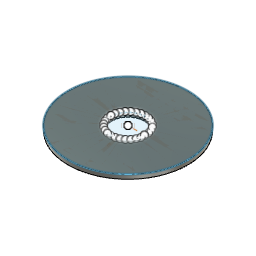
Untitled v1 (Autodesk Fusion 360 design; units mm, degrees)
Autodesk Fusion 360 part; units mm, degrees
sketch "Sketch2" plane through (0, 0, 0) normal (0, 0, 1) x (1, 0, 0)
  circle A0 centre (0, 0) radius 139.7
  dimension "d37" = 279.4
  constraint coincident A0.centre origin
  measures "d37" diameter of A0
sketch "Sketch1" plane through (0, 0, 0) normal (0, 0, 1) x (1, 0, 0)
  circle A0 centre (0, 0) radius 139.7
  line L0 (7.734, 37.3068) -> (8.2303, 39.481)
  line L1 (9.2198, 36.9676) -> (9.7161, 39.1418)
  line L2 (15.8416, 34.6505) -> (16.8092, 36.6597)
  line L3 (17.2146, 33.9892) -> (18.1823, 35.9985)
  line L4 (23.1548, 30.2567) -> (24.5452, 32.0003)
  line L5 (24.3463, 29.3065) -> (25.7367, 31.05)
  line L6 (29.3069, 24.3457) -> (31.0505, 25.7362)
  line L7 (30.2571, 23.1542) -> (32.0007, 24.5447)
  line L8 (33.9895, 17.214) -> (35.9988, 18.1816)
  line L9 (34.6507, 15.841) -> (36.66, 16.8086)
  line L10 (36.9678, 9.2192) -> (39.142, 9.7154)
  line L11 (37.3069, 7.7334) -> (39.4811, 8.2296)
  line L12 (-0.7493, 40.3155) -> (-0.7493, 38.0926)
  line L13 (0.7493, 40.3155) -> (0.7493, 38.0926)
  arc A1 (15.8416, 34.6505) -> (9.2198, 36.9676) centre (0, 0) ccw
  arc A2 (23.1548, 30.2567) -> (17.2146, 33.9892) centre (0, 0) ccw
  arc A3 (18.1791, 35.992) -> (16.8061, 36.6532) centre (0, 0) ccw
  arc A4 (25.7322, 31.0444) -> (24.5407, 31.9946) centre (0, 0) ccw
  arc A5 (31.9951, 24.5402) -> (31.0449, 25.7317) centre (0, 0) ccw
  arc A6 (29.3069, 24.3457) -> (24.3463, 29.3065) centre (0, 0) ccw
  arc A7 (36.6535, 16.8054) -> (35.9923, 18.1785) centre (0, 0) ccw
  arc A8 (33.9895, 17.214) -> (30.2571, 23.1542) centre (0, 0) ccw
  arc A9 (36.9678, 9.2192) -> (34.6507, 15.841) centre (0, 0) ccw
  arc A10 (39.4741, 8.228) -> (39.135, 9.7138) centre (0, 0) ccw
  arc A11 (38.0926, 0.7493) -> (37.3069, 7.7334) centre (0, 0) ccw
  line L14 (38.0926, 0.7493) -> (40.3155, 0.7493)
  line L15 (38.0926, -0.7493) -> (40.3155, -0.7493)
  arc A12 (9.7145, 39.1348) -> (8.2287, 39.4739) centre (0, 0) ccw
  line L16 (7.734, -37.3068) -> (8.2303, -39.481)
  arc A13 (8.2287, -39.4739) -> (9.7145, -39.1348) centre (0, 0) ccw
  line L17 (9.2198, -36.9676) -> (9.7161, -39.1418)
  arc A14 (9.2198, -36.9676) -> (15.8416, -34.6505) centre (0, 0) ccw
  line L18 (15.8416, -34.6505) -> (16.8092, -36.6597)
  arc A15 (16.8061, -36.6532) -> (18.1791, -35.992) centre (0, 0) ccw
  line L19 (17.2146, -33.9892) -> (18.1823, -35.9985)
  arc A16 (17.2146, -33.9892) -> (23.1548, -30.2567) centre (0, 0) ccw
  line L20 (23.1548, -30.2567) -> (24.5452, -32.0003)
  arc A17 (24.5407, -31.9946) -> (25.7322, -31.0444) centre (0, 0) ccw
  line L21 (24.3463, -29.3065) -> (25.7367, -31.05)
  arc A18 (24.3463, -29.3065) -> (29.3069, -24.3457) centre (0, 0) ccw
  line L22 (29.3069, -24.3457) -> (31.0505, -25.7362)
  arc A19 (31.0449, -25.7317) -> (31.9951, -24.5402) centre (0, 0) ccw
  line L23 (30.2571, -23.1542) -> (32.0007, -24.5447)
  arc A20 (30.2571, -23.1542) -> (33.9895, -17.214) centre (0, 0) ccw
  line L24 (33.9895, -17.214) -> (35.9988, -18.1816)
  arc A21 (35.9923, -18.1785) -> (36.6535, -16.8054) centre (0, 0) ccw
  line L25 (34.6507, -15.841) -> (36.66, -16.8086)
  arc A22 (34.6507, -15.841) -> (36.9678, -9.2192) centre (0, 0) ccw
  line L26 (36.9678, -9.2192) -> (39.142, -9.7154)
  arc A23 (39.135, -9.7138) -> (39.4741, -8.228) centre (0, 0) ccw
  line L27 (37.3069, -7.7334) -> (39.4811, -8.2296)
  arc A24 (37.3069, -7.7334) -> (38.0926, -0.7493) centre (0, 0) ccw
  line L28 (0, 0) -> (38.1, 0) construction
  arc A25 (40.3155, -0.7493) -> (40.3155, 0.7493) centre (0, 0) ccw
  arc A26 (18.1791, 35.992) -> (16.8061, 36.6532) centre (0, 0) ccw
  arc A27 (25.7322, 31.0444) -> (24.5407, 31.9946) centre (0, 0) ccw
  arc A28 (31.9951, 24.5402) -> (31.0449, 25.7317) centre (0, 0) ccw
  arc A29 (39.4741, 8.228) -> (39.135, 9.7138) centre (0, 0) ccw
  arc A30 (36.6535, 16.8054) -> (35.9923, 18.1785) centre (0, 0) ccw
  arc A31 (9.7145, 39.1348) -> (8.2287, 39.4739) centre (0, 0) ccw
  arc A32 (39.135, -9.7138) -> (39.4741, -8.228) centre (0, 0) ccw
  arc A33 (35.9923, -18.1785) -> (36.6535, -16.8054) centre (0, 0) ccw
  arc A34 (31.0449, -25.7317) -> (31.9951, -24.5402) centre (0, 0) ccw
  arc A35 (24.5407, -31.9946) -> (25.7322, -31.0444) centre (0, 0) ccw
  arc A36 (16.8061, -36.6532) -> (18.1791, -35.992) centre (0, 0) ccw
  arc A37 (8.2287, -39.4739) -> (9.7145, -39.1348) centre (0, 0) ccw
  arc A38 (34.6507, -15.841) -> (36.9678, -9.2192) centre (0, 0) ccw
  arc A39 (30.2571, -23.1542) -> (33.9895, -17.214) centre (0, 0) ccw
  arc A40 (24.3463, -29.3065) -> (29.3069, -24.3457) centre (0, 0) ccw
  arc A41 (17.2146, -33.9892) -> (23.1548, -30.2567) centre (0, 0) ccw
  arc A42 (9.2198, -36.9676) -> (15.8416, -34.6505) centre (0, 0) ccw
  arc A43 (-40.3155, 0.7493) -> (-40.3155, -0.7493) centre (0, 0) ccw
  line L29 (-38.0926, -0.7493) -> (-40.3155, -0.7493)
  arc A44 (-38.0926, -0.7493) -> (-37.3069, -7.7334) centre (0, 0) ccw
  line L30 (-37.3069, -7.7334) -> (-39.4811, -8.2296)
  line L31 (-34.6507, -15.841) -> (-36.66, -16.8086)
  arc A45 (-39.4741, -8.228) -> (-39.135, -9.7138) centre (0, 0) ccw
  line L32 (-36.9678, -9.2192) -> (-39.142, -9.7154)
  arc A46 (-36.9678, -9.2192) -> (-34.6507, -15.841) centre (0, 0) ccw
  arc A47 (-36.6535, -16.8054) -> (-35.9923, -18.1785) centre (0, 0) ccw
  line L33 (-33.9895, -17.214) -> (-35.9988, -18.1816)
  arc A48 (-33.9895, -17.214) -> (-30.2571, -23.1542) centre (0, 0) ccw
  line L34 (-30.2571, -23.1542) -> (-32.0007, -24.5447)
  arc A49 (-31.9951, -24.5402) -> (-31.0449, -25.7317) centre (0, 0) ccw
  line L35 (-29.3069, -24.3457) -> (-31.0505, -25.7362)
  arc A50 (-29.3069, -24.3457) -> (-24.3463, -29.3065) centre (0, 0) ccw
  line L36 (-24.3463, -29.3065) -> (-25.7367, -31.05)
  arc A51 (-25.7322, -31.0444) -> (-24.5407, -31.9946) centre (0, 0) ccw
  line L37 (-23.1548, -30.2567) -> (-24.5452, -32.0003)
  arc A52 (-23.1548, -30.2567) -> (-17.2146, -33.9892) centre (0, 0) ccw
  arc A53 (-18.1791, -35.992) -> (-16.8061, -36.6532) centre (0, 0) ccw
  line L38 (-17.2146, -33.9892) -> (-18.1823, -35.9985)
  line L39 (-15.8416, -34.6505) -> (-16.8092, -36.6597)
  arc A54 (-15.8416, -34.6505) -> (-9.2198, -36.9676) centre (0, 0) ccw
  line L40 (-9.2198, -36.9676) -> (-9.7161, -39.1418)
  arc A55 (-9.7145, -39.1348) -> (-8.2287, -39.4739) centre (0, 0) ccw
  line L41 (-7.734, -37.3068) -> (-8.2303, -39.481)
  arc A56 (-15.8416, -34.6505) -> (-9.2198, -36.9676) centre (0, 0) ccw
  arc A57 (-15.8416, -34.6505) -> (-9.2198, -36.9676) centre (0, 0) ccw
  arc A58 (-0.7493, -40.3155) -> (0.7493, -40.3155) centre (0, 0) ccw
  arc A59 (-9.7145, -39.1348) -> (-8.2287, -39.4739) centre (0, 0) ccw
  arc A60 (-0.7493, -40.3155) -> (0, -40.3225) centre (0, 0) ccw
  arc A61 (-9.7145, -39.1348) -> (-8.2287, -39.4739) centre (0, 0) ccw
  arc A62 (-18.1791, -35.992) -> (-16.8061, -36.6532) centre (0, 0) ccw
  arc A63 (-18.1791, -35.992) -> (-16.8061, -36.6532) centre (0, 0) ccw
  arc A64 (-25.7322, -31.0444) -> (-24.5407, -31.9946) centre (0, 0) ccw
  arc A65 (-36.6535, -16.8054) -> (-35.9923, -18.1785) centre (0, 0) ccw
  arc A66 (-39.4741, -8.228) -> (-39.135, -9.7138) centre (0, 0) ccw
  arc A67 (-39.4741, -8.228) -> (-39.135, -9.7138) centre (0, 0) ccw
  arc A68 (-31.9951, -24.5402) -> (-31.0449, -25.7317) centre (0, 0) ccw
  arc A69 (-25.7322, -31.0444) -> (-24.5407, -31.9946) centre (0, 0) ccw
  arc A70 (-23.1548, -30.2567) -> (-17.2146, -33.9892) centre (0, 0) ccw
  arc A71 (-29.3069, -24.3457) -> (-24.3463, -29.3065) centre (0, 0) ccw
  arc A72 (-24.3463, -29.3065) -> (-17.2146, -33.9892) centre (0, 0) ccw
  arc A73 (-33.9895, -17.214) -> (-30.2571, -23.1542) centre (0, 0) ccw
  arc A74 (-36.6535, -16.8054) -> (-35.9923, -18.1785) centre (0, 0) ccw
  arc A75 (-31.9951, -24.5402) -> (-31.0449, -25.7317) centre (0, 0) ccw
  arc A76 (-36.9678, -9.2192) -> (-34.6507, -15.841) centre (0, 0) ccw
  arc A77 (-36.9678, -9.2192) -> (-34.6507, -15.841) centre (0, 0) ccw
  arc A78 (-33.9895, -17.214) -> (-30.2571, -23.1542) centre (0, 0) ccw
  arc A79 (-38.0926, -0.7493) -> (-37.3069, -7.7334) centre (0, 0) ccw
  arc A80 (-38.0926, -0.7493) -> (-37.3069, -7.7334) centre (0, 0) ccw
  arc A81 (-7.734, -37.3068) -> (-0.7493, -38.0926) centre (0, 0) ccw
  arc A82 (-7.734, -37.3068) -> (-0.7493, -38.0926) centre (0, 0) ccw
  arc A83 (0.762, -38.0924) -> (7.734, -37.3068) centre (0, 0) ccw
  arc A84 (-7.734, -37.3068) -> (-0.7493, -38.0926) centre (0, 0) ccw
  arc A85 (0.762, -38.0924) -> (7.734, -37.3068) centre (0, 0) ccw
  line L42 (0.762, -38.0924) -> (0.7493, -40.3155)
  line L43 (-0.7493, -38.0926) -> (-0.7493, -40.3155)
  arc A86 (15.8416, 34.6505) -> (9.2198, 36.9676) centre (0, 0) ccw
  arc A87 (15.8416, 34.6505) -> (9.2198, 36.9676) centre (0, 0) ccw
  arc A88 (23.1548, 30.2567) -> (17.2146, 33.9892) centre (0, 0) ccw
  arc A89 (23.1548, 30.2567) -> (17.2146, 33.9892) centre (0, 0) ccw
  arc A90 (29.3069, 24.3457) -> (24.3463, 29.3065) centre (0, 0) ccw
  arc A91 (29.3069, 24.3457) -> (24.3463, 29.3065) centre (0, 0) ccw
  arc A92 (33.9895, 17.214) -> (30.2571, 23.1542) centre (0, 0) ccw
  arc A93 (33.9895, 17.214) -> (30.2571, 23.1542) centre (0, 0) ccw
  arc A94 (36.9678, 9.2192) -> (34.6507, 15.841) centre (0, 0) ccw
  arc A95 (38.0926, 0.7493) -> (37.3069, 7.7334) centre (0, 0) ccw
  arc A96 (36.9678, 9.2192) -> (34.6507, 15.841) centre (0, 0) ccw
  arc A97 (38.0926, 0.7493) -> (37.3069, 7.7334) centre (0, 0) ccw
  line L44 (-40.3155, 0.7493) -> (-38.0926, 0.7493)
  arc A98 (0, 40.3225) -> (-0.7493, 40.3155) centre (0, 0) ccw
  line L45 (-0.7493, 38.0926) -> (-0.7493, 40.3155)
  arc A99 (-0.7493, 38.0926) -> (-7.734, 37.3068) centre (0, 0) ccw
  line L46 (-7.734, 37.3068) -> (-8.2303, 39.481)
  arc A100 (-8.2287, 39.4739) -> (-9.7145, 39.1348) centre (0, 0) ccw
  line L47 (-9.2198, 36.9676) -> (-9.7161, 39.1418)
  arc A101 (-9.2198, 36.9676) -> (-15.8416, 34.6505) centre (0, 0) ccw
  line L48 (-15.8416, 34.6505) -> (-16.8092, 36.6597)
  arc A102 (-16.8061, 36.6532) -> (-18.1791, 35.992) centre (0, 0) ccw
  line L49 (-17.2146, 33.9892) -> (-18.1823, 35.9985)
  arc A103 (-17.2146, 33.9892) -> (-23.1548, 30.2567) centre (0, 0) ccw
  line L50 (-23.1548, 30.2567) -> (-24.5452, 32.0003)
  line L51 (-24.3463, 29.3065) -> (-25.7367, 31.05)
  arc A104 (-24.5407, 31.9946) -> (-25.7322, 31.0444) centre (0, 0) ccw
  arc A105 (-24.3463, 29.3065) -> (-29.3069, 24.3457) centre (0, 0) ccw
  line L52 (-29.3069, 24.3457) -> (-31.0505, 25.7362)
  arc A106 (-31.0449, 25.7317) -> (-31.9951, 24.5402) centre (0, 0) ccw
  line L53 (-30.2571, 23.1542) -> (-32.0007, 24.5447)
  line L54 (-33.9895, 17.214) -> (-35.9988, 18.1816)
  arc A107 (-35.9923, 18.1785) -> (-36.6535, 16.8054) centre (0, 0) ccw
  line L55 (-34.6507, 15.841) -> (-36.66, 16.8086)
  arc A108 (-34.6507, 15.841) -> (-36.9678, 9.2192) centre (0, 0) ccw
  line L56 (-36.9678, 9.2192) -> (-39.142, 9.7154)
  arc A109 (-39.135, 9.7138) -> (-39.4741, 8.228) centre (0, 0) ccw
  line L57 (-37.3069, 7.7334) -> (-39.4811, 8.2296)
  arc A110 (-37.3069, 7.7334) -> (-38.0926, 0.7493) centre (0, 0) ccw
  line L58 (-38.0926, 0.7493) -> (-40.3155, 0.7493)
  arc A111 (-40.3155, 0.7493) -> (-40.3155, -0.7493) centre (0, 0) ccw
  arc A112 (0.7493, 40.3155) -> (-0.7493, 40.3155) centre (0, 0) ccw
  arc A113 (-31.0449, 25.7317) -> (-31.9951, 24.5402) centre (0, 0) ccw
  arc A114 (-24.5407, 31.9946) -> (-25.7322, 31.0444) centre (0, 0) ccw
  arc A115 (-16.8061, 36.6532) -> (-18.1791, 35.992) centre (0, 0) ccw
  arc A116 (-24.5407, 31.9946) -> (-25.7322, 31.0444) centre (0, 0) ccw
  arc A117 (-8.2287, 39.4739) -> (-9.7145, 39.1348) centre (0, 0) ccw
  arc A118 (-16.8061, 36.6532) -> (-18.1791, 35.992) centre (0, 0) ccw
  arc A119 (0.7493, 40.3155) -> (-0.7493, 40.3155) centre (0, 0) ccw
  arc A120 (-8.2287, 39.4739) -> (-9.7145, 39.1348) centre (0, 0) ccw
  arc A121 (7.734, 37.3068) -> (0.7493, 38.0926) centre (0, 0) ccw
  arc A122 (-9.2198, 36.9676) -> (-15.8416, 34.6505) centre (0, 0) ccw
  arc A123 (-17.2146, 33.9892) -> (-23.1548, 30.2567) centre (0, 0) ccw
  arc A124 (-31.0449, 25.7317) -> (-31.9951, 24.5402) centre (0, 0) ccw
  arc A125 (-35.9923, 18.1785) -> (-36.6535, 16.8054) centre (0, 0) ccw
  arc A126 (-40.3155, 0.7493) -> (-40.3155, -0.7493) centre (0, 0) ccw
  arc A127 (-35.9923, 18.1785) -> (-36.6535, 16.8054) centre (0, 0) ccw
  arc A128 (-39.135, 9.7138) -> (-39.4741, 8.228) centre (0, 0) ccw
  arc A129 (-39.135, 9.7138) -> (-39.4741, 8.228) centre (0, 0) ccw
  arc A130 (-40.3155, 0.7493) -> (-40.3155, -0.7493) centre (0, 0) ccw
  arc A131 (-37.3069, 7.7334) -> (-38.0926, 0.7493) centre (0, 0) ccw
  arc A132 (-37.3069, 7.7334) -> (-38.0926, 0.7493) centre (0, 0) ccw
  arc A133 (-24.3463, 29.3065) -> (-29.3069, 24.3457) centre (0, 0) ccw
  arc A134 (-30.2571, 23.1542) -> (-33.9895, 17.214) centre (0, 0) ccw
  arc A135 (-34.6507, 15.841) -> (-36.9678, 9.2192) centre (0, 0) ccw
  arc A136 (-34.6507, 15.841) -> (-36.9678, 9.2192) centre (0, 0) ccw
  arc A137 (-37.3069, 7.7334) -> (-38.0926, 0.7493) centre (0, 0) ccw
  arc A138 (-24.3463, 29.3065) -> (-29.3069, 24.3457) centre (0, 0) ccw
  arc A139 (-9.2198, 36.9676) -> (-15.8416, 34.6505) centre (0, 0) ccw
  arc A140 (-17.2146, 33.9892) -> (-23.1548, 30.2567) centre (0, 0) ccw
  arc A141 (-0.7493, 38.0926) -> (-7.734, 37.3068) centre (0, 0) ccw
  arc A142 (-9.2198, 36.9676) -> (-15.8416, 34.6505) centre (0, 0) ccw
  arc A143 (7.734, 37.3068) -> (0.7493, 38.0926) centre (0, 0) ccw
  arc A144 (-0.7493, 38.0926) -> (-7.734, 37.3068) centre (0, 0) ccw
  arc A145 (7.734, 37.3068) -> (0.7493, 38.0926) centre (0, 0) ccw
  arc A146 (-0.7493, 38.0926) -> (-7.734, 37.3068) centre (0, 0) ccw
  arc A147 (37.3069, -7.7334) -> (38.0926, -0.7493) centre (0, 0) ccw
  arc A148 (34.6507, -15.841) -> (36.9678, -9.2192) centre (0, 0) ccw
  arc A149 (30.2571, -23.1542) -> (33.9895, -17.214) centre (0, 0) ccw
  arc A150 (24.3463, -29.3065) -> (29.3069, -24.3457) centre (0, 0) ccw
  arc A151 (17.2146, -33.9892) -> (23.1548, -30.2567) centre (0, 0) ccw
  arc A152 (0.762, -38.0924) -> (7.734, -37.3068) centre (0, 0) ccw
  arc A153 (9.2198, -36.9676) -> (15.8416, -34.6505) centre (0, 0) ccw
  dimension "d38" = 279.4
  constraint coincident L12.start A3
  constraint coincident L13.start A3
  constraint coincident L2.start A143
  constraint coincident L4.start A143
  constraint coincident L6.start A143
  constraint coincident L8.start A143
  constraint coincident L10.start A143
  constraint coincident A11.start A143
  constraint coincident L12.end A143
  constraint concentric A1 A143
  constraint concentric A2 A143
  constraint coincident L4 A4.end
  constraint coincident L3 A3.start
  constraint coincident L2 A3.end
  constraint coincident L1 A12.start
  constraint concentric A3 A12
  constraint coincident L6 A5.end
  constraint coincident L5 A4.start
  constraint concentric A4 A12
  constraint coincident L8 A7.end
  constraint coincident L7 A5.start
  constraint concentric A5 A12
  constraint concentric A6 A143
  constraint coincident L10 A10.end
  constraint coincident L9 A7.start
  constraint concentric A7 A12
  constraint concentric A8 A143
  constraint concentric A9 A143
  constraint coincident L11 A10.start
  constraint concentric A10 A12
  constraint concentric A11 A143
  constraint coincident L15.end A12
  constraint coincident L0 A12.end
  constraint concentric A12 A112
  constraint concentric A25 A29
  constraint concentric A29 A31
  constraint concentric A26 A29
  constraint concentric A27 A29
  constraint concentric A28 A29
  constraint concentric A29 A30
  constraint concentric A31 A119
  constraint concentric A32 A112
  constraint concentric A33 A112
  constraint concentric A34 A112
  constraint concentric A35 A112
  constraint concentric A36 A112
  constraint concentric A37 A112
  constraint concentric A38 A143
  constraint concentric A39 A143
  constraint concentric A40 A143
  constraint concentric A41 A143
  constraint concentric A42 A143
  constraint concentric A82 A143
  constraint concentric A57 A95
  constraint concentric A56 A143
  constraint concentric A57 A84
  constraint concentric A58 A119
  constraint concentric A59 A119
  constraint concentric A60 A112
  constraint concentric A61 A112
  constraint concentric A62 A112
  constraint concentric A63 A119
  constraint concentric A64 A119
  constraint concentric A68 A112
  constraint concentric A74 A119
  constraint concentric A65 A112
  constraint concentric A66 A112
  constraint concentric A67 A119
  constraint concentric A68 A69
  constraint concentric A70 A95
  constraint concentric A71 A95
  constraint concentric A72 A143
  constraint concentric A73 A95
  constraint concentric A74 A75
  constraint concentric A77 A143
  constraint concentric A76 A95
  constraint concentric A77 A78
  constraint concentric A79 A143
  constraint concentric A80 A95
  constraint concentric A81 A152
  constraint concentric A82 A83
  constraint concentric A84 A85
  constraint concentric A121 A152
  constraint concentric A86 A95
  constraint concentric A86 A145
  constraint concentric A87 A152
  constraint concentric A88 A152
  constraint concentric A89 A95
  constraint concentric A90 A95
  constraint concentric A91 A152
  constraint concentric A92 A95
  constraint concentric A93 A152
  constraint concentric A94 A152
  constraint concentric A95 A96
  constraint concentric A97 A152
  constraint concentric A112 A117
  constraint concentric A115 A119
  constraint concentric A114 A117
  constraint concentric A113 A115
  constraint concentric A113 A127
  constraint concentric A139 A143
  constraint concentric A121 A133
  constraint concentric A134 A139
  constraint concentric A114 A124
  constraint concentric A115 A116
  constraint concentric A117 A118
  constraint concentric A119 A120
  constraint concentric A121 A141
  constraint concentric A122 A145
  constraint concentric A123 A141
  constraint concentric A124 A125
  constraint concentric A125 A129
  constraint concentric A126 A127
  constraint concentric A127 A128
  constraint concentric A129 A130
  constraint concentric A132 A134
  constraint concentric A133 A136
  constraint concentric A134 A135
  constraint concentric A136 A137
  constraint concentric A138 A139
  measures "d38" diameter of A0
extrude "Extrude1" add sketch "Sketch1" against normal blind 10.1854
equation "E0_P_OD_IN = 11 in" comment "if E0_P_OD_IN >7:; E0_P_OD_IN = E0_P_OD_IN;else:;  E0_P_OD_IN=11;"
equation "E0_P_ID_IN = 3.0 in"
equation "E0_P_T1_IN = 0.4010 in"
equation "E0_P_M_IN = 12.857 deg"
equation "E0_P_ID2_IN = 3.175 in"
equation "E0_P_A1_IN = 0.03 in"
equation "d35 = -E0_P_T1_IN"
equation "d37 = E0_P_OD_IN"
equation "d38 = E0_P_OD_IN"
